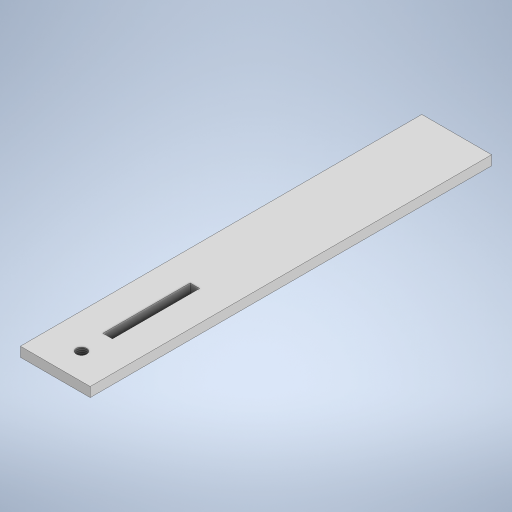
# Autodesk Inventor part: LMK
Saved by Autodesk Inventor 2023 (Build 270158000, 158)
## iProperties
Created: 2022-10-24
Part Number: LMK
Material: Generic
Document SubType Name: Modeling
Designer: User
Density: 1 g/cm^3
Appearance: Default
Author: User
Autodesk Inventor part; units mm, degrees
ref_plane "YZ Plane" through (0, 0, 0) normal (1, 0, 0) x (0, 1, 0)
ref_plane "XZ Plane" through (0, 0, 0) normal (0, 1, 0) x (-1, 0, 0)
ref_plane "XY Plane" through (0, 0, 0) normal (0, 0, 1) x (1, 0, 0)
sketch "Sketch1" plane through (0, 0, 0) normal (0, 1, 0) x (-1, 0, 0)
  line L0 (0, 0) -> (0, -230)
  line L1 (0, -230) -> (40, -230)
  line L2 (40, -230) -> (40, 0)
  line L3 (40, 0) -> (0, 0)
  dimension "d0" = 230
  dimension "d1" = 40
  constraints: 8 end point, 3 perpendicular, 1 vertical
  measures "d0" distance of L0.start L0.end
  measures "d1" distance of L0.end L1.end
extrude "Extrusion1" add sketch "Sketch1" along normal blind 5.5
sketch "Sketch2" plane through (0, 5.5, 0) normal (0, 1, 0) x (1, 0, 0)
  line L0 (-40, 0) -> (0, 0) construction
  line L1 (-20, 0) -> (-20, 30) construction
  line L2 (-20, 30) -> (-22.75, 30)
  line L3 (-40, 230) -> (-40, 0) construction
  line L4 (-22.75, 30) -> (-22.75, 80)
  line L5 (-22.75, 80) -> (-20, 80)
  line L6 (-20, 30) -> (-17.25, 30)
  line L7 (-17.25, 30) -> (-17.25, 80)
  line L8 (-17.25, 80) -> (-20, 80)
  dimension "d4" = 30
  dimension "d5" = 2.75
  dimension "d6" = 50
  constraints: 14 end point, 2 symmetric about line, 2 vertical, 1 horizontal, 1 midpoint, 1 perpendicular
  measures "d4" distance of L1.start L1.end
  measures "d5" distance of L1.end L2.end
  measures "d6" distance of L2.end L4.end
extrude "Extrusion2" cut sketch "Sketch2" against normal blind 5.5
sketch "Sketch3" plane through (0, 5.5, 0) normal (0, 1, 0) x (1, 0, 0)
  line L0 (-40, 0) -> (0, 0) construction
  line L1 (-20, 0) -> (-20, 15) construction
  dimension "d9" = 15
  constraints: 2 end point, 1 coincident, 1 midpoint, 1 vertical
  measures "d9" distance of L1.start L1.end
hole "Hole1" at (-20, 5.5, -15) direction (0, -1, 0) diameter 5.9175 depth 19.1 tip angle 118 thread size "M7x1" class "6H" standard "ANSI Metric M Profile"
body "Solid1"
